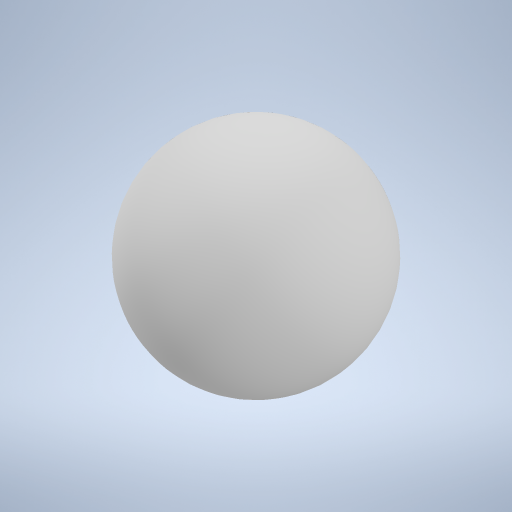
# Autodesk Inventor part: wheel_simplified
Saved by Autodesk Inventor 2023 (Build 270158000, 158)
## iProperties
Created: 2022-08-10
Part Number: wheel_simplified
Material: Genérico
Document SubType Name: Modeling
Designer: victo
Density: 1 g/cm^3
Appearance: Padrão
Author: victo
Autodesk Inventor part; units mm, degrees
ref_plane "YZ Plane" through (0, 0, 0) normal (1, 0, 0) x (0, 1, 0)
ref_plane "XZ Plane" through (0, 0, 0) normal (0, 1, 0) x (-1, 0, 0)
ref_plane "XY Plane" through (0, 0, 0) normal (0, 0, 1) x (1, 0, 0)
sketch "Esboço1" plane through (0, 0, 0) normal (0, 0, 1) x (1, 0, 0)
  line L0 (-24.75, 0) -> (24.75, 0)
  circle A0 centre (0, 0) radius 24.75
  dimension "d0" = 49.5
  constraints: 2 end point, 2 point on circle, 1 centre point, 1 coincident, 1 horizontal
  measures "d0" diameter of A0
revolve "Revolução1" add sketch "Esboço1" angle 360 about axis through (-24.75, 0, 0) along (1, 0, 0) picked at (-2.9255, -7.7139) contours L0 A0
